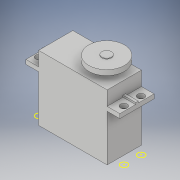
# Autodesk Inventor part: FS5106B_servo
Saved by Autodesk Inventor 2018 (Build 220112000, 112)
## iProperties
Created: 2018-04-21
Part Number: FS5106B_servo
Material: Generic
Document SubType Name: Modeling
Designer: scwu
Density: 1 g/cm^3
Appearance: Default
Author: scwu
Autodesk Inventor part; units mm, degrees
ref_plane "YZ Plane" through (0, 0, 0) normal (1, 0, 0) x (0, 1, 0)
ref_plane "XZ Plane" through (0, 0, 0) normal (0, 1, 0) x (-1, 0, 0)
ref_plane "XY Plane" through (0, 0, 0) normal (0, 0, 1) x (1, 0, 0)
sketch "Sketch1" plane through (0, 0, 0) normal (0, 0, 1) x (1, 0, 0)
  line L0 (-20, 0) -> (20, 0)
  line L1 (20, 0) -> (20, 27.1)
  line L2 (20, 27.1) -> (27.4, 27.1)
  line L3 (27.4, 27.1) -> (27.4, 29.6)
  line L4 (27.4, 29.6) -> (20, 29.6)
  line L5 (20, 29.6) -> (20, 37.9)
  line L6 (20, 37.9) -> (-20, 37.9)
  line L7 (-20, 37.9) -> (-20, 29.6)
  line L8 (-20, 29.6) -> (-27.4, 29.6)
  line L9 (-27.4, 29.6) -> (-27.4, 27.1)
  line L10 (-27.4, 27.1) -> (-20, 27.1)
  line L11 (-20, 27.1) -> (-20, 0)
  point P0 (0, 0)
  point P1 (0, 0)
  dimension "d0" = 40
  dimension "d1" = 27.1
  dimension "d2" = 7.4
  dimension "d3" = 2.5
  dimension "d4" = 8.3
  dimension "d5" = 7.4
  constraints: 24 end point, 9 perpendicular, 3 point on line, 2 horizontal, 1 coincident, 1 midpoint
  measures "d0" distance of L0.start L0.end
  measures "d1" distance of L0.end L1.end
  measures "d2" distance of L1.end L2.end
  measures "d3" distance of L2.end L3.end
  measures "d4" distance of L4.end L5.end
  measures "d5" distance of L7.end L8.end
extrude "Extrusion1" add sketch "Sketch1" along normal mid plane 20
sketch "Sketch4" plane through (0, 0, 0) normal (0, 0, 1) x (1, 0, 0)
  line L0 (20, 37.9) -> (-20, 37.9) projected
  line L1 (12.5, 37.9) -> (12.5, 42.3)
  line L2 (12.5, 42.3) -> (20.1, 42.3)
  line L3 (20.1, 42.3) -> (20.1, 45.3)
  line L4 (20.1, 45.3) -> (12.5, 45.3)
  line L5 (12.5, 45.3) -> (12.5, 45.7)
  line L6 (12.5, 45.7) -> (9.7, 45.7)
  line L7 (12.5, 37.9) -> (9.7, 37.9)
  line L8 (9.7, 45.7) -> (9.7, 37.9)
  point P0 (0, 0)
  point P1 (0, 37.9)
  dimension "d10" = 9.7
  dimension "d11" = 0.4
  dimension "d12" = 10.4
  dimension "d13" = 2.8
  dimension "d14" = 4.4
  dimension "d15" = 3
  constraints: 16 end point, 4 perpendicular, 4 point on line, 2 vertical, 1 midpoint
  measures "d10" distance from line of L8 point (0, 37.9)
  measures "d11" distance of L4.end L5.end
  measures "d12" distance between parallel lines of L3 L8
  measures "d13" distance between parallel lines of L8 L1
  measures "d14" distance of L1.start L1.end
  measures "d15" distance of L2.end L3.end
revolve "Revolution1" add sketch "Sketch4" angle 360 about axis through (9.7, 45.7, 0) along (0, -1, 0)
sketch "Sketch5" plane through (-27.4, 29.6, 10) normal (0, 1, 0) x (1, 0, 0)
  circle A0 centre (2.65, 15) radius 2
  line L0 (0, 20) -> (0, 0) projected
  line L1 (7.4, 0) -> (0, 0) projected
  line L2 (7.4, 20) -> (7.4, 0) projected
  line L3 (0, 20) -> (7.4, 20) projected
  line L4 (47.4, 20) -> (47.4, 0) projected
  line L5 (54.8, 0) -> (47.4, 0) projected
  line L6 (54.8, 20) -> (54.8, 0) projected
  line L7 (47.4, 20) -> (54.8, 20) projected
  line L8 (7.4, 20) -> (47.4, 20) projected
  line L9 (27.4, 20) -> (27.4, 0) construction
  line L10 (7.4, 0) -> (47.4, 0) projected
  line L11 (0, 20) -> (0, 0) projected
  line L12 (0, 10) -> (54.8, 10) construction
  line L13 (54.8, 20) -> (54.8, 0) projected
  circle A1 centre (2.65, 5) radius 2
  circle A2 centre (52.15, 15) radius 2
  circle A3 centre (52.15, 5) radius 2
  line L14 (7.4, 0) -> (7.4, 20) projected
  line L15 (7.4, 10.75) -> (0, 10.75)
  line L16 (0, 10.75) -> (0, 9.25)
  line L17 (0, 9.25) -> (7.4, 9.25)
  line L18 (7.4, 9.25) -> (7.4, 10.75)
  line L19 (47.4, 10.75) -> (54.8, 10.75)
  line L20 (54.8, 10.75) -> (54.8, 9.25)
  line L21 (54.8, 9.25) -> (47.4, 9.25)
  line L22 (47.4, 9.25) -> (47.4, 10.75)
  point P0 (27.4, 10)
  dimension "d17" = 4
  dimension "d18" = 10
  dimension "d19" = 49.5
  dimension "d22" = 7.4
  dimension "d23" = 1.5
  constraints: 20 end point, 7 symmetric about line, 4 centre point, 4 midpoint, 2 parallel, 1 horizontal, 1 perpendicular, 1 point on line, 4 other
  measures "d17" diameter of A0
  measures "d18" distance of A1.centre A0.centre
  measures "d19" distance of A0.centre A2.centre
  measures "d22" distance of L17.end L16.end
  measures "d23" distance of L16.end L15.end
extrude "Extrusion2" cut sketch "Sketch5" against normal up to next contours A0 | A1 | A2 | A3
extrude "Extrusion3" add sketch "Sketch5" along normal blind 1 contours L15 L2 L17 L0 | L19 L6 L21 L4
sketch "Sketch6" plane through (-20, 0, 10) normal (0, -1, 0) x (1, 0, 0)
  line L0 (0, 0) -> (0, -20) construction
  line L1 (0, -10) -> (40, -10) construction
  line L2 (40, -20) -> (40, 0) construction
  line L3 (40, 0) -> (0, 0) construction
  line L4 (20, 0) -> (20, -20) construction
  line L5 (0, -20) -> (40, -20) construction
  line L6 (40, 0) -> (0, 0) construction
  line L7 (0, 0) -> (0, -20) construction
  line L8 (0, -20) -> (40, -20) construction
  line L9 (40, -20) -> (40, 0) construction
  circle A0 centre (29.7, -10) radius 2.8 projected
  circle A1 centre (-4.75, -5) radius 2 projected
  circle A2 centre (-4.75, -15) radius 2 projected
  circle A3 centre (44.75, -15) radius 2 projected
  circle A4 centre (44.75, -5) radius 2 projected
  point P0 (20, -10)
  point P1 (29.7, -10)
  constraints: 12 end point, 4 midpoint, 2 parallel, 1 coincident, 1 horizontal, 1 perpendicular
body "Solid1"
